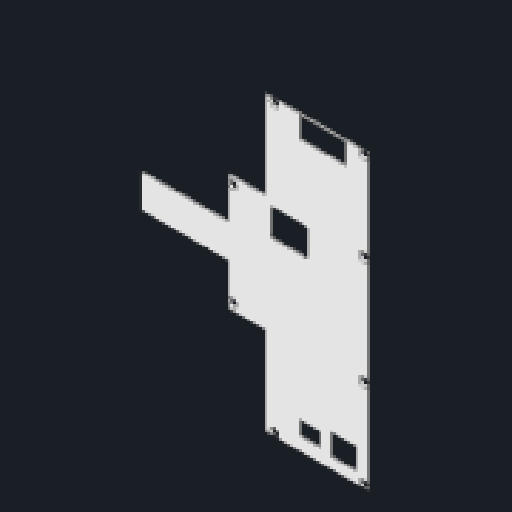
# Autodesk Inventor part: ceil
Saved by Autodesk Inventor 2023 (Build 270158000, 158)
## iProperties
Created: 2024-05-26
Part Number: ceil
Material: ABS Plastic
Document SubType Name: Modeling
Designer: szymo
Density: 1.06 g/cm^3
Appearance: Smooth - White
Mass: 13.4096 g
Surface Area: 263.221 cm^2
Volume: 12.6506 cm^3
Author: szymo
Autodesk Inventor part; units mm, degrees
ref_plane "YZ Plane" through (0, 0, 0) normal (1, 0, 0) x (0, 1, 0)
ref_plane "XZ Plane" through (0, 0, 0) normal (0, 1, 0) x (-1, 0, 0)
ref_plane "XY Plane" through (0, 0, 0) normal (0, 0, 1) x (1, 0, 0)
sketch "Sketch1" plane through (0, 0, 0) normal (0, 0, 1) x (1, 0, 0)
  arc A0 (81.0648, -49.5) -> (80.0648, -50.5) centre (81.0648, -50.5) ccw projected
  line L0 (80.0648, -52.5) -> (80.0648, -50.5) projected
  line L1 (35, -52.5) -> (80.0648, -52.5) projected
  line L2 (35, -52.5) -> (35, -50.5) projected
  arc A1 (30, -45.5) -> (35, -50.5) centre (35, -45.5) ccw projected
  line L3 (30, -45.5) -> (30, -37.5) projected
  line L4 (22.4833, -37.5) -> (30, -37.5) projected
  line L5 (22.4833, -47.5) -> (22.4833, -37.5) projected
  arc A2 (17.4833, -52.5) -> (22.4833, -47.5) centre (17.4833, -47.5) ccw projected
  line L6 (12.5167, -52.5) -> (17.4833, -52.5) projected
  arc A3 (7.5167, -47.5) -> (12.5167, -52.5) centre (12.5167, -47.5) ccw projected
  line L7 (7.5167, -47.5) -> (7.5167, -37.5) projected
  line L8 (0, -37.5) -> (7.5167, -37.5) projected
  line L9 (0, -53.5) -> (0, -37.5) projected
  line L10 (85.0648, -53.5) -> (0, -53.5) projected
  line L11 (85.0648, -53.5) -> (85.0648, -49.8187) projected
  arc A4 (85.0648, -49.8187) -> (84.3327, -49.5) centre (84.3327, -50.5) ccw projected
  line L12 (81.0648, -49.5) -> (84.3327, -49.5) projected
  circle A5 centre (82.5648, -51.5) radius 1.75 projected
  circle A6 centre (28, -51.5) radius 1.75 projected
  arc A7 (80.0648, 121.5) -> (81.0648, 120.5) centre (81.0648, 121.5) ccw projected
  line L13 (81.0648, 120.5) -> (84.3327, 120.5) projected
  arc A8 (84.3327, 120.5) -> (85.0648, 120.8187) centre (84.3327, 121.5) ccw projected
  line L14 (85.0648, 124.5) -> (85.0648, 120.8187) projected
  line L15 (85.0648, 124.5) -> (0, 124.5) projected
  line L16 (0, 124.5) -> (0, 108.5) projected
  line L17 (0, 108.5) -> (7.5167, 108.5) projected
  line L18 (7.5167, 118.5) -> (7.5167, 108.5) projected
  arc A9 (12.5167, 123.5) -> (7.5167, 118.5) centre (12.5167, 118.5) ccw projected
  line L19 (12.5167, 123.5) -> (17.4833, 123.5) projected
  arc A10 (22.4833, 118.5) -> (17.4833, 123.5) centre (17.4833, 118.5) ccw projected
  line L20 (22.4833, 118.5) -> (22.4833, 108.5) projected
  line L21 (22.4833, 108.5) -> (30, 108.5) projected
  line L22 (30, 116.5) -> (30, 108.5) projected
  arc A11 (35, 121.5) -> (30, 116.5) centre (35, 116.5) ccw projected
  line L23 (35, 123.5) -> (35, 121.5) projected
  line L24 (35, 123.5) -> (80.0648, 123.5) projected
  line L25 (80.0648, 123.5) -> (80.0648, 121.5) projected
  circle A12 centre (82.5648, 122.5) radius 1.75 projected
  circle A13 centre (28, 122.5) radius 1.75 projected
  line L26 (70.3148, 112) -> (70.3148, 123) projected
  line L27 (70.3148, 123) -> (44.3148, 123) projected
  line L28 (44.3148, 123) -> (44.3148, 112) projected
  line L29 (44.3148, 112) -> (70.3148, 112) projected
  line L30 (76.5648, -34.9) -> (63.5648, -34.9) projected
  line L31 (63.5648, -34.9) -> (63.5648, -45.9) projected
  line L32 (63.5648, -45.9) -> (76.5648, -45.9) projected
  line L33 (76.5648, -45.9) -> (76.5648, -34.9) projected
  line L34 (55.0648, -37.9) -> (44.5648, -37.9) projected
  line L35 (44.5648, -37.9) -> (44.5648, -44.4) projected
  line L36 (44.5648, -44.4) -> (55.0648, -44.4) projected
  line L37 (55.0648, -44.4) -> (55.0648, -37.9) projected
  arc A14 (-1, 24.3) -> (0, 25.3) centre (-1, 25.3) ccw projected
  line L38 (5.352, 25.3) -> (0, 25.3) projected
  line L39 (5.352, 28.3) -> (5.352, 25.3) projected
  line L40 (-52.5, 28.3) -> (5.352, 28.3) projected
  line L41 (-52.5, 28.3) -> (-52.5, 24.3) projected
  line L42 (-46.5, 24.3) -> (-52.5, 24.3) projected
  arc A15 (-46.5, 24.3) -> (-45.5, 25.3) centre (-46.5, 25.3) ccw projected
  line L43 (-7, 25.3) -> (-45.5, 25.3) projected
  arc A16 (-7, 25.3) -> (-6, 24.3) centre (-6, 25.3) ccw projected
  line L44 (-1, 24.3) -> (-6, 24.3) projected
  arc A17 (0, 45.7) -> (-1, 46.7) centre (-1, 45.7) ccw projected
  line L45 (-1, 46.7) -> (-6, 46.7) projected
  arc A18 (-6, 46.7) -> (-7, 45.7) centre (-6, 45.7) ccw projected
  line L46 (-7, 45.7) -> (-45.5, 45.7) projected
  arc A19 (-45.5, 45.7) -> (-46.5, 46.7) centre (-46.5, 45.7) ccw projected
  line L47 (-46.5, 46.7) -> (-52.5, 46.7) projected
  line L48 (-52.5, 42.7) -> (-52.5, 46.7) projected
  line L49 (-52.5, 42.7) -> (5.352, 42.7) projected
  line L50 (5.352, 42.7) -> (5.352, 45.7) projected
  line L51 (5.352, 45.7) -> (0, 45.7) projected
  line L52 (0, 124.5) -> (85.0648, 124.5)
  line L53 (85.0648, 124.5) -> (85.0648, -53.5)
  line L54 (85.0648, -53.5) -> (0, -53.5)
  line L55 (0, -53.5) -> (0, 124.5)
  line L56 (0, 5.7) -> (0, 65.3)
  line L57 (-52.5, 65.3) -> (-52.5, 5.7)
  line L58 (0, 5.7) -> (0, 8.7)
  line L59 (-52.5, 8.7) -> (-52.5, 5.7)
  line L60 (0, 45.7) -> (-52.5, 45.7)
  line L61 (-52.5, 45.7) -> (-52.5, 42.7)
  line L62 (-52.5, 42.7) -> (0, 42.7)
  line L63 (0, 42.7) -> (0, 45.7)
  line L64 (0, 65.3) -> (-52.5, 65.3)
  line L65 (-52.5, 65.3) -> (-52.5, 62.3)
  line L66 (0, 62.3) -> (0, 65.3)
  line L67 (-52.5, 28.3) -> (0, 28.3)
  line L68 (0, 28.3) -> (0, 25.3)
  line L69 (0, 25.3) -> (-52.5, 25.3)
  line L70 (-52.5, 25.3) -> (-52.5, 28.3)
  line L71 (-52.5, 28.3) -> (0, 28.3)
  line L72 (0, 28.3) -> (0, 42.7)
  line L73 (0, 42.7) -> (-52.5, 42.7)
  line L74 (-52.5, 42.7) -> (-52.5, 28.3)
  line L75 (43.5648, -36.9) -> (56.0648, -36.9)
  line L76 (56.0648, -36.9) -> (56.0648, -45.4)
  line L77 (56.0648, -45.4) -> (43.5648, -45.4)
  line L78 (43.5648, -45.4) -> (43.5648, -36.9)
  line L79 (62.5648, -46.9) -> (62.5648, -33.9)
  line L80 (62.5648, -33.9) -> (77.5648, -33.9)
  line L81 (77.5648, -33.9) -> (77.5648, -46.9)
  line L82 (77.5648, -46.9) -> (62.5648, -46.9)
  line L83 (43.3148, 111) -> (43.3148, 124)
  line L84 (43.3148, 124) -> (71.3148, 124)
  line L85 (71.3148, 124) -> (71.3148, 111)
  line L86 (71.3148, 111) -> (43.3148, 111)
  line L87 (26.9124, 51.3) -> (47.4124, 51.3) projected
  ellipse E0 centre (26.9117, 51.3993) end of major axis (26.9821, 51.3289) minor radius 0.099 (26.8124, 51.4) -> (26.9124, 51.3) ccw projected
  line L88 (26.8124, 65.9) -> (26.8124, 51.4) projected
  ellipse E1 centre (26.9117, 65.9007) end of major axis (26.9821, 65.9711) minor radius 0.099 (26.9124, 66) -> (26.8124, 65.9) ccw projected
  ellipse E2 centre (47.4131, 51.3993) end of major axis (47.4835, 51.4697) minor radius 0.099 (47.4124, 51.3) -> (47.5124, 51.4) ccw projected
  line L89 (47.5124, 51.4) -> (47.5124, 65.9) projected
  ellipse E3 centre (47.4131, 65.9007) end of major axis (47.4835, 65.8303) minor radius 0.099 (47.5124, 65.9) -> (47.4124, 66) ccw projected
  line L90 (48.5124, 65.9001) -> (48.5124, 51.3999)
  line L91 (47.4125, 50.3) -> (26.9123, 50.3)
  line L92 (25.8124, 51.3999) -> (25.8124, 65.9001)
  line L93 (26.9123, 67) -> (47.4125, 67)
  circle A20 centre (2.676, 66.65) radius 1.75 projected
  circle A21 centre (82.5648, 68.5) radius 1.75 projected
  line L94 (85.0648, 71) -> (-3.5, 71) projected
  line L95 (-3.5, 71) -> (-49, 71) projected
  line L96 (-49, 71) -> (-52.5, 71) projected
  line L97 (-52.5, 71) -> (-52.5, 64.3) projected
  line L98 (-52.5, 64.3) -> (5.352, 64.3) projected
  line L99 (5.352, 64.5) -> (5.352, 64.3) projected
  arc A22 (6.852, 66) -> (5.352, 64.5) centre (6.852, 64.5) ccw projected
  line L100 (6.852, 66) -> (85.0648, 66) projected
  line L101 (85.0648, 71) -> (85.0648, 66) projected
  line L102 (-12.0597, 0) -> (-10.0597, 0) projected
  circle A23 centre (2.676, 4.35) radius 1.75 projected
  circle A24 centre (82.5648, 2.5) radius 1.75 projected
  line L103 (85.0648, 0) -> (-3.5, 0) projected
  line L104 (85.0648, 0) -> (85.0648, 5) projected
  line L105 (6.852, 5) -> (85.0648, 5) projected
  arc A25 (5.352, 6.5) -> (6.852, 5) centre (6.852, 6.5) ccw projected
  line L106 (5.352, 6.5) -> (5.352, 6.7) projected
  line L107 (-52.5, 6.7) -> (5.352, 6.7) projected
  line L108 (-52.5, 0) -> (-52.5, 6.7) projected
  line L109 (-49, 0) -> (-52.5, 0) projected
  line L110 (-3.5, 0) -> (-49, 0) projected
  line L111 (0, -53.5) -> (22.4833, -53.5)
  line L112 (22.4833, -53.5) -> (22.4833, 0)
  line L113 (22.4833, 0) -> (0, 0)
  line L114 (0, 0) -> (0, -53.5)
  line L115 (0, 71) -> (22.4833, 71)
  line L116 (22.4833, 71) -> (22.4833, 124.5)
  line L117 (22.4833, 124.5) -> (0, 124.5)
  line L118 (0, 124.5) -> (0, 71)
  spline S0 degree 5 poles (47.4125, 67) (47.7581, 67.0001) (48.1038, 66.8645) (48.3769, 66.5914) (48.5125, 66.2457) (48.5124, 65.9001) knots 0 0 0 0 0 0 1 1 1 1 1 1
  spline S1 degree 5 poles (48.5124, 51.3999) (48.5125, 51.0543) (48.3769, 50.7086) (48.1038, 50.4355) (47.7581, 50.2999) (47.4125, 50.3) knots 0 0 0 0 0 0 1 1 1 1 1 1
  spline S2 degree 5 poles (26.9123, 50.3) (26.5667, 50.2999) (26.221, 50.4355) (25.9479, 50.7086) (25.8123, 51.0543) (25.8124, 51.3999) knots 0 0 0 0 0 0 1 1 1 1 1 1
  spline S3 degree 5 poles (25.8124, 65.9001) (25.8123, 66.2457) (25.9479, 66.5914) (26.221, 66.8645) (26.5667, 67.0001) (26.9123, 67) knots 0 0 0 0 0 0 1 1 1 1 1 1
  point P0 (43.3148, 123.5)
  point P1 (71.3148, 123.5)
  point P2 (0, 25.3)
  point P3 (0, 45.7)
  point P4 (-7, 45.7)
  point P5 (0, 28.3)
  point P6 (0, 25.3)
  point P7 (85.0648, -49.8187)
  point P8 (-7, 25.3)
  point P9 (0, 45.7)
  point P10 (-7, 45.7)
  point P11 (0, 25.3)
  dimension "d12" = 1
  dimension "d0" = 1
  dimension "d1" = 1
  dimension "d2" = 1
  constraints: 94 end point, 21 parallel, 8 horizontal, 7 perpendicular, 7 point on line, 25 other
  measures "d0" distance between parallel lines of L34 L75
  measures "d1" distance between parallel lines of L31 L79
  measures "d2" distance between parallel lines of L28 L83
extrude "Extrusion1" add sketch "Sketch1" along normal blind 1 contours L12 A4 L11 L10 L112 L5 L4 L3 A1 L2 L1 L0 A0 | A0 L0 L1 L2 A1 L3 L4 L112 L103 L53 A4 L12 | L103 L55 L107 L106 A25 L105 L53 | L105 A25 L106 L107 L55 L38 L39 L40 L49 L50 L51 L98 L99 A22 L100 S3 L92 S2 L91 S1 L90 S0 L53 | L100 S0 L93 S3 A22 L99 L98 L55 L94 L53 | L94 L116 L21 L22 A11 L23 L24 L83 L86 L85 L25 A7 L13 A8 L53 | A8 L13 A7 L25 L24 L85 L84 L83 L23 A11 L22 L21 L20 L116 L15 L14 | L55 L40 L39 L38 | L69 L43 L41 L40 L55 | L40 L57 L49 L55 | L55 L51 L50 L49 | L49 L48 L60 L46 L55 | L24 L83 L84 L85 | A5 | A6 | A12 | A13 | A20 | A21 | A23 | A24
sketch "Sketch2" plane through (0, 0, 1) normal (0, 0, 1) x (1, 0, 0)
  arc A0 (81.0648, -49.5) -> (80.0648, -50.5) centre (81.0648, -50.5) ccw projected
  line L0 (80.0648, -52.5) -> (80.0648, -50.5) projected
  line L1 (35, -52.5) -> (80.0648, -52.5) projected
  line L2 (35, -52.5) -> (35, -50.5) projected
  arc A1 (30, -45.5) -> (35, -50.5) centre (35, -45.5) ccw projected
  line L3 (30, -45.5) -> (30, -37.5) projected
  line L4 (22.4833, -37.5) -> (30, -37.5) projected
  line L5 (22.4833, -47.5) -> (22.4833, -37.5) projected
  arc A2 (17.4833, -52.5) -> (22.4833, -47.5) centre (17.4833, -47.5) ccw projected
  line L6 (12.5167, -52.5) -> (17.4833, -52.5) projected
  arc A3 (7.5167, -47.5) -> (12.5167, -52.5) centre (12.5167, -47.5) ccw projected
  line L7 (7.5167, -47.5) -> (7.5167, -37.5) projected
  line L8 (0, -37.5) -> (7.5167, -37.5) projected
  line L9 (0, -53.5) -> (0, -37.5) projected
  line L10 (85.0648, -53.5) -> (0, -53.5) projected
  line L11 (85.0648, -53.5) -> (85.0648, -49.8187) projected
  arc A4 (85.0648, -49.8187) -> (84.3327, -49.5) centre (84.3327, -50.5) ccw projected
  line L12 (81.0648, -49.5) -> (84.3327, -49.5) projected
  circle A5 centre (82.5648, -51.5) radius 1.75 projected
  circle A6 centre (28, -51.5) radius 1.75 projected
  circle A7 centre (2.676, 4.35) radius 1.75 projected
  circle A8 centre (82.5648, 2.5) radius 1.75 projected
  line L13 (0, 0) -> (85.0648, 0) projected
  line L14 (85.0648, 0) -> (85.0648, 5) projected
  line L15 (12.4976, 5) -> (85.0648, 5) projected
  arc A9 (5.352, 8.7) -> (12.4976, 5) centre (12.4976, 13.75) ccw projected
  line L16 (-52.5, 8.7) -> (5.352, 8.7) projected
  line L17 (-52.5, 5.7) -> (-52.5, 8.7) projected
  line L18 (-52.5, 5.7) -> (-49, 5.7) projected
  line L19 (-49, 5.7) -> (-3.5, 5.7) projected
  line L20 (-3.5, 5.7) -> (-2.1566, 5.7) projected
  arc A10 (-1.2313, 5.0793) -> (-2.1566, 5.7) centre (-2.1566, 4.7) ccw projected
  arc A11 (0, 0) -> (-1.2313, 5.0793) centre (-17.28, -1.5) ccw projected
  arc A12 (80.0648, 121.5) -> (81.0648, 120.5) centre (81.0648, 121.5) ccw projected
  line L21 (81.0648, 120.5) -> (84.3327, 120.5) projected
  arc A13 (84.3327, 120.5) -> (85.0648, 120.8187) centre (84.3327, 121.5) ccw projected
  line L22 (85.0648, 124.5) -> (85.0648, 120.8187) projected
  line L23 (85.0648, 124.5) -> (0, 124.5) projected
  line L24 (0, 124.5) -> (0, 108.5) projected
  line L25 (0, 108.5) -> (7.5167, 108.5) projected
  line L26 (7.5167, 118.5) -> (7.5167, 108.5) projected
  arc A14 (12.5167, 123.5) -> (7.5167, 118.5) centre (12.5167, 118.5) ccw projected
  line L27 (12.5167, 123.5) -> (17.4833, 123.5) projected
  arc A15 (22.4833, 118.5) -> (17.4833, 123.5) centre (17.4833, 118.5) ccw projected
  line L28 (22.4833, 118.5) -> (22.4833, 108.5) projected
  line L29 (22.4833, 108.5) -> (30, 108.5) projected
  line L30 (30, 116.5) -> (30, 108.5) projected
  arc A16 (35, 121.5) -> (30, 116.5) centre (35, 116.5) ccw projected
  line L31 (35, 123.5) -> (35, 121.5) projected
  line L32 (35, 123.5) -> (80.0648, 123.5) projected
  line L33 (80.0648, 123.5) -> (80.0648, 121.5) projected
  circle A17 centre (82.5648, 122.5) radius 1.75 projected
  circle A18 centre (28, 122.5) radius 1.75 projected
  circle A19 centre (2.676, 66.65) radius 1.75 projected
  circle A20 centre (82.5648, 68.5) radius 1.75 projected
  line L34 (85.0648, 71) -> (-3.5, 71) projected
  line L35 (-3.5, 71) -> (-49, 71) projected
  line L36 (-49, 71) -> (-52.5, 71) projected
  line L37 (-52.5, 71) -> (-52.5, 64.3) projected
  line L38 (-52.5, 64.3) -> (5.352, 64.3) projected
  line L39 (5.352, 64.5) -> (5.352, 64.3) projected
  arc A21 (6.852, 66) -> (5.352, 64.5) centre (6.852, 64.5) ccw projected
  line L40 (6.852, 66) -> (85.0648, 66) projected
  line L41 (85.0648, 71) -> (85.0648, 66) projected
  point P0 (82.5648, 68.5)
  point P1 (2.676, 66.65)
  constraints: 6 coincident
hole "Hole1" at (82.5648, -51.5, 1) at (28, -51.5, 1) at (2.676, 4.35, 1) at (82.5648, 2.5, 1) at (82.5648, 68.5, 1) at (2.676, 66.65, 1) at (82.5648, 122.5, 1) at (28, 122.5, 1) direction (0, 0, -1) diameter 2.9 end through all countersink diameter 5.5 countersink angle 90 clearance for "Countersunk Flat Head Screw ISO 2009/7046" size "M2.5" standard "ISO"
body "Solid1"
